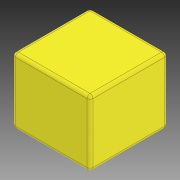
# Autodesk Inventor part: Power Cube
Saved by Autodesk Inventor 2021 (Build 250183000, 183)
## iProperties
Created: 2020-10-27
Part Number: Power Cube
Material: Generic
Document SubType Name: Modeling
Density: 1 g/cm^3
Appearance: Canary
Autodesk Inventor part; units mm, degrees
ref_plane "YZ Plane" through (0, 0, 0) normal (1, 0, 0) x (0, 1, 0)
ref_plane "XZ Plane" through (0, 0, 0) normal (0, 1, 0) x (-1, 0, 0)
ref_plane "XY Plane" through (0, 0, 0) normal (0, 0, 1) x (1, 0, 0)
sketch "Sketch1" plane through (0, 0, 0) normal (0, 1, 0) x (-1, 0, 0)
  line L0 (-165.1, -165.1) -> (165.1, -165.1)
  line L1 (165.1, -165.1) -> (165.1, 165.1)
  line L2 (165.1, 165.1) -> (-165.1, 165.1)
  line L3 (-165.1, 165.1) -> (-165.1, -165.1)
  line L4 (-165.1, -165.1) -> (165.1, 165.1) construction
  line L5 (165.1, -165.1) -> (-165.1, 165.1) construction
  point P0 (0, 0)
  dimension "d0" = 330.2
  dimension "d1" = 330.2
  constraints: 12 end point, 2 midpoint, 2 parallel, 1 horizontal, 1 perpendicular
  measures "d0" distance of L2.end L1.end
  measures "d1" distance of L1.end L0.end
extrude "Extrusion1" add sketch "Sketch1" along normal mid plane 279.4
fillet "Fillet1" radius 12.7 12 edges at (-165.1, -139.7, 0) (0, -139.7, -165.1) (165.1, -139.7, 0) (0, -139.7, 165.1) (-165.1, 0, -165.1) (0, 139.7, -165.1) (165.1, 0, -165.1) (165.1, 139.7, 0) (165.1, 0, 165.1) (0, 139.7, 165.1) (-165.1, 0, 165.1) (-165.1, 139.7, 0)
body "Solid1"
